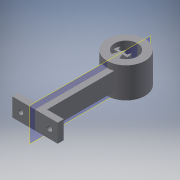
# Autodesk Inventor part: frontSight
Saved by Autodesk Inventor 2018 (Build 220112000, 112)
## iProperties
Created: 2017-11-07
Part Number: frontSight
Material: Generic
Document SubType Name: Modeling
Designer: Prakash
Density: 1 g/cm^3
Appearance: Default
Author: Prakash
Autodesk Inventor part; units mm, degrees
note: some values were not read from the file. Chosen so that the rebuilt part matches the saved one: direction of "Hole1".
ref_plane "YZ Plane" through (0, 0, 0) normal (1, 0, 0) x (0, 1, 0)
ref_plane "XZ Plane" through (0, 0, 0) normal (0, 1, 0) x (-1, 0, 0)
ref_plane "XY Plane" through (0, 0, 0) normal (0, 0, 1) x (1, 0, 0)
sketch "Sketch1" plane through (0, 0, 0) normal (0, 0, 1) x (1, 0, 0)
  line L0 (0, 0) -> (30, 0)
  line L1 (30, 0) -> (30, 4)
  line L2 (30, 4) -> (0, 4)
  line L3 (0, 4) -> (0, 0)
  line L4 (15, 4) -> (11, 4)
  line L5 (15, 4) -> (19, 4)
  line L6 (11, 4) -> (11, 60)
  line L7 (19, 4) -> (19, 60)
  line L8 (11, 60) -> (19, 60)
  circle A0 centre (15, 60) radius 7.5
  circle A1 centre (15, 60) radius 12.5
  arc A2 (11, 48.1573) -> (19, 48.1573) centre (15, 60) ccw
  arc A3 (11, 53.6557) -> (19, 53.6557) centre (15, 60) ccw
  dimension "d0" = 30
  dimension "d1" = 4
  dimension "d2" = 4
  dimension "d3" = 4
  dimension "d5" = 60
  dimension "d6" = 15
  dimension "d7" = 25
  constraints: 18 end point, 8 point on circle, 6 point on line, 4 centre point, 3 parallel, 2 concentric, 2 horizontal, 2 midpoint, 2 vertical, 1 coincident, 1 perpendicular
  measures "d0" distance of L2.end L1.end
  measures "d1" distance of L1.end L0.end
  measures "d2" distance of L4.start L4.end
  measures "d3" distance of L4.start L5.end
  measures "d5" distance from line of L0 L6.end
  measures "d6" diameter of A0
  measures "d7" diameter of A1
extrude "Extrusion1" add sketch "Sketch1" along normal mid plane 12 contours L3 L2 L1 L0 | L6 A1 L7 L2
extrude "Extrusion2" add sketch "Sketch1" along normal mid plane 20 contours A1 L7 A0 L6 | L6 A0 L7 A1
sketch "Sketch2" plane through (19, 4, 6) normal (0, 1, 0) x (1, 0, 0)
  line L0 (0, 12) -> (0, 0) projected
  line L1 (11, 0) -> (0, 0) projected
  line L2 (11, 12) -> (11, 0) projected
  line L3 (0, 12) -> (11, 12) projected
  line L4 (0, 6) -> (11, 6)
  point P0 (-19, 6)
  point P1 (5.5, 6)
  constraints: 3 midpoint, 2 end point
hole "Hole1" at (24.5, 4, 0) direction (0, -1, 0) diameter 3.5 end up to surface
ref_plane "Work Plane1" through (15, 4, -6) normal (-1, 0, 0) x (0, 0, 1)
mirror "Mirror1" about plane through (15, 4, -6) normal (-1, 0, 0) of "Hole1"
sketch "Sketch3" plane through (15, 60, 10) normal (0, 0, 1) x (1, 0, 0)
  circle A0 centre (0, 0) radius 7.5 projected
  line L0 (0, 0) -> (2.5652, -7.0477)
  line L1 (0, 0) -> (-2.5652, -7.0477)
  line L2 (0, -74.5) -> (0, 27) projected
  line L3 (0, -7.5) -> (0, -2.25)
  line L4 (0, 0) -> (-7.5, 0)
  line L5 (7.5, 0) -> (0, 0)
  line L6 (3.75, 0) -> (4.5689, -2.25)
  line L7 (0, -3.75) -> (4.5689, -3.75)
  line L8 (4.5689, -3.75) -> (4.5689, -2.25)
  line L9 (2.9311, -2.25) -> (0, -2.25)
  line L10 (0, -2.25) -> (0, -3.75)
  line L11 (3.75, 0) -> (2.9311, -2.25)
  arc A1 (-2.5652, -7.0477) -> (2.5652, -7.0477) centre (0, 0) ccw
  point P0 (-15, -60)
  point P1 (-3.75, 0)
  dimension "d19" = 20
  dimension "d20" = 20
  dimension "d21" = 70
  dimension "d22" = 1.5
  dimension "d23" = 70
  dimension "d24" = 4.5689
  dimension "d25" = 2.9311
  constraints: 23 end point, 8 point on circle, 2 horizontal, 2 midpoint, 2 parallel, 2 perpendicular, 2 point on line, 1 centre point, 1 collinear
  measures "d19" angle of L2 L0
  measures "d20" angle of L2 L1
  measures "d21" angle of L5 L6
  measures "d22" distance of L6.end L7.end
  measures "d23" angle of L5 L11
  measures "d24" distance of L7.start L7.end
  measures "d25" distance of L9.start L3.end
extrude "Extrusion3" add sketch "Sketch3" against normal up to surface (20 mm away) contours L1 L2 A0 | L0 L9 L2 | L2 L7 L0 A0 | L9 L11 L6 L8 L7 L0 | L0 L7 L2 L9
mirror "Mirror2" about plane through (15, 4, -6) normal (-1, 0, 0) of "Extrusion3"
equation "\"d2\" = d3"
equation "\"d20\" = d19"
equation "\"d23\" = d21"
body "Solid1"
